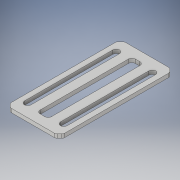
# Autodesk Inventor part: Holder
Saved by Autodesk Inventor 2019 (Build 230136000, 136)
## iProperties
Created: 2019-03-24
Part Number: Holder
Material: Ogólny
Document SubType Name: Modeling
Designer: atmat
Density: 1 g/cm^3
Appearance: Domyślna
Author: atmat
Autodesk Inventor part; units mm, degrees
ref_plane "YZ Plane" through (0, 0, 0) normal (1, 0, 0) x (0, 1, 0)
ref_plane "XZ Plane" through (0, 0, 0) normal (0, 1, 0) x (-1, 0, 0)
ref_plane "XY Plane" through (0, 0, 0) normal (0, 0, 1) x (1, 0, 0)
sketch "Szkic1" plane through (0, 0, 0) normal (0, 1, 0) x (-1, 0, 0)
  line L0 (14, 30) -> (-14, 30)
  line L1 (-14, 30) -> (-14, -30)
  line L2 (-14, -30) -> (14, -30)
  line L3 (14, -30) -> (14, 30)
  point P0 (0, 0)
  dimension "d0" = 28
  dimension "d1" = 14
  dimension "d2" = 60
  dimension "d3" = 30
  constraints: 8 end point, 2 parallel, 1 horizontal, 1 perpendicular
  measures "d0" distance of L0.start L0.end
  measures "d1" distance from line of point (0, 0) L3
  measures "d2" distance of L2.end L0.start
  measures "d3" distance from line of point (0, 0) L2
extrude "Wyciągnięcie proste1" add sketch "Szkic1" along normal blind 2
sketch "Szkic2" plane through (0, 2, 0) normal (0, 1, 0) x (1, 0, 0)
  line L0 (-11.25, -25) -> (-7.75, -25)
  line L1 (-7.75, -25) -> (-7.75, 25)
  line L2 (-7.75, 25) -> (-11.25, 25)
  line L3 (-11.25, 25) -> (-11.25, -25)
  line L4 (7.75, -25) -> (11.25, -25)
  line L5 (11.25, -25) -> (11.25, 25)
  line L6 (11.25, 25) -> (7.75, 25)
  line L7 (7.75, 25) -> (7.75, -25)
  line L8 (-14, -30) -> (14, -30) projected
  line L9 (14, 30) -> (-14, 30) projected
  point P0 (0, 0)
  dimension "d6" = 3.5
  dimension "d7" = 3.5
  dimension "d8" = 5
  dimension "d9" = 0
  dimension "d10" = 5
  dimension "d11" = 0
  dimension "d12" = 15.5
  dimension "d13" = 7.75
  constraints: 16 end point, 4 parallel, 2 horizontal, 2 perpendicular
  measures "d6" distance between parallel lines of L5 L7
  measures "d7" distance between parallel lines of L1 L3
  measures "d8" distance between parallel lines of L8 L0
  measures "d9" distance between parallel lines of L0 L4
  measures "d10" distance between parallel lines of L9 L2
  measures "d11" distance between parallel lines of L2 L6
  measures "d12" distance between parallel lines of L7 L1
  measures "d13" distance from line of point (0, 0) L1
extrude "Wyciągnięcie proste2" cut sketch "Szkic2" against normal blind 2
chamfer "Faza1" distance 2 angle 45 4 edges at (-14, 1, 30) (-14, 1, -30) (14, 1, -30) (14, 1, 30)
sketch "Szkic3" plane through (0, 2, 0) normal (0, 1, 0) x (1, 0, 0)
  line L0 (-3, -25) -> (3, -25)
  line L1 (3, -25) -> (3, 25)
  line L2 (3, 25) -> (-3, 25)
  line L3 (-3, 25) -> (-3, -25)
  point P0 (0, 0)
  dimension "d19" = 50
  dimension "d20" = 25
  dimension "d21" = 6
  dimension "d22" = 3
  constraints: 8 end point, 2 parallel, 1 horizontal, 1 perpendicular
  measures "d19" distance of L0.end L1.end
  measures "d20" distance from line of point (0, 0) L2
  measures "d21" distance of L1.end L2.end
  measures "d22" distance from line of point (0, 0) L3
extrude "Wyciągnięcie proste3" cut sketch "Szkic3" against normal blind 2
fillet "Zaokrąglenie1" radius 1.75 12 edges at (3, 1, 25) (-7.75, 1, 25) (-11.25, 1, 25) (-3, 1, 25) (7.75, 1, 25) (-11.25, 1, -25) (-7.75, 1, -25) (-3, 1, -25) (3, 1, -25) (7.75, 1, -25) (11.25, 1, -25) (11.25, 1, 25)
fillet "Zaokrąglenie2" radius 1.75 8 edges at (-12, 1, -30) (-14, 1, -28) (12, 1, -30) (14, 1, -28) (12, 1, 30) (14, 1, 28) (-12, 1, 30) (-14, 1, 28)
